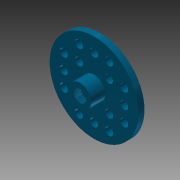
# Autodesk Inventor part: 13-0002
Saved by Autodesk Inventor 2015 SP1 (Build 190203100, 203)
## iProperties
Category: Servo Kit
Company: Autodesk Inc.
Created: 2014-11-30
Part Number: 13-0002
Material: Polystyrene, High Impact
Document SubType Name: Modeling
Designer: Matrix
Density: 1.022 g/cm^3
Appearance: Sky Blue Dark
Catalog Web Link: http://matrixrobotics.com/
Vendor: Matrix
Author: Autodesk Inc.
Autodesk Inventor part; units mm, degrees
ref_plane "YZ Plane" through (0, 0, 0) normal (1, 0, 0) x (0, 1, 0)
ref_plane "XZ Plane" through (0, 0, 0) normal (0, 1, 0) x (-1, 0, 0)
sketch "Sketch1" plane through (0, 0, 0) normal (0, 1, 0) x (-1, 0, 0)
  circle A0 centre (0, 0) radius 6
  circle A1 centre (0, 0) radius 23.5
  circle A2 centre (8, -8) radius 2.1
  circle A3 centre (-8, -8) radius 2.1
  circle A4 centre (7.961966, 8) radius 2.1
  circle A5 centre (-8, 8) radius 2.1
  circle A6 centre (0, 16) radius 2.1
  circle A7 centre (16, 8) radius 2.1
  circle A8 centre (16, -8) radius 2.1
  circle A9 centre (0, -16) radius 2.1
  circle A10 centre (-16, -8) radius 2.1
  circle A11 centre (-16, 8) radius 2.1
  circle A12 centre (0, 0) radius 3
  circle A13 centre (-16, 0) radius 2.1
  circle A14 centre (-8, -16) radius 2.1
  circle A15 centre (8, -16) radius 2.1
  circle A16 centre (16, 0) radius 2.1
  circle A17 centre (8, 16) radius 2.1
  circle A18 centre (-8, 16) radius 2.1
  constraints: 19 centre point
extrude "Extrusion1" add sketch "Sketch1" against normal blind 3.2 contours A0 | A1 | A12
extrude "Extrusion2" add sketch "Sketch1" along normal blind 7.5 contours A0 | A12
sketch "Sketch2" plane through (0, 7.5, 0) normal (0, 1, 0) x (1, 0, 0)
  line L0 (0.096605, 3.117984) -> (0.054534, 3.057901)
  arc A0 (-0.937297, 2.916297) -> (-1.313083, 2.767513) centre (-1.085967, 2.74284) ccw
  line L1 (-0.937297, 2.916297) -> (-0.881604, 2.868563)
  arc A1 (-0.881604, 2.868563) -> (-0.609384, 2.938457) centre (-0.769964, 2.998815) ccw
  line L2 (-0.609384, 2.938457) -> (-0.583576, 3.007117)
  arc A2 (-0.182595, 3.057773) -> (-0.583576, 3.007117) centre (-0.369732, 2.926739) ccw
  line L3 (-0.182595, 3.057773) -> (-0.140524, 2.997689)
  arc A3 (-0.140524, 2.997689) -> (0.140525, 2.997689) centre (0.000001, 3.096085) ccw
  line L4 (0.140525, 2.997689) -> (0.182596, 3.057773)
  arc A4 (0.583577, 3.007117) -> (0.182596, 3.057773) centre (0.369733, 2.926738) ccw
  line L5 (0.583577, 3.007117) -> (0.609385, 2.938457)
  arc A5 (0.609385, 2.938457) -> (0.881605, 2.868563) centre (0.769965, 2.998815) ccw
  line L6 (0.881605, 2.868563) -> (0.937297, 2.916297)
  arc A6 (1.313083, 2.767513) -> (0.937297, 2.916297) centre (1.085967, 2.74284) ccw
  line L7 (1.313083, 2.767513) -> (1.321005, 2.694592)
  arc A7 (1.321005, 2.694592) -> (1.56729, 2.559195) centre (1.49155, 2.713119) ccw
  line L8 (1.56729, 2.559195) -> (1.633105, 2.59158)
  arc A8 (1.960083, 2.354016) -> (1.633105, 2.59158) centre (1.733967, 2.3866) ccw
  line L9 (1.960083, 2.354016) -> (1.949622, 2.281416)
  arc A9 (1.949622, 2.281416) -> (2.154499, 2.089025) centre (2.119417, 2.256948) ccw
  line L10 (2.154499, 2.089025) -> (2.226295, 2.104024)
  arc A10 (2.483923, 1.792608) -> (2.226295, 2.104024) centre (2.273014, 1.880401) ccw
  line L11 (2.483923, 1.792608) -> (2.455735, 1.724891)
  arc A11 (2.455735, 1.724891) -> (2.606329, 1.487593) centre (2.614111, 1.658965) ccw
  line L12 (2.606329, 1.487593) -> (2.679603, 1.484265)
  arc A12 (2.851689, 1.118563) -> (2.679603, 1.484265) centre (2.66924, 1.256049) ccw
  line L13 (2.851689, 1.118563) -> (2.807546, 1.059983)
  arc A13 (2.807546, 1.059983) -> (2.894395, 0.792689) centre (2.944551, 0.956742) ccw
  line L14 (2.894395, 0.792689) -> (2.964538, 0.771244)
  arc A14 (3.040272, 0.374235) -> (2.964538, 0.771244) centre (2.897746, 0.552775) ccw
  line L15 (3.040272, 0.374235) -> (2.982949, 0.328474)
  arc A15 (2.982949, 0.328474) -> (3.000596, 0.047979) centre (3.089974, 0.194405) ccw
  line L16 (3.000596, 0.047979) -> (3.063204, 0.009763)
  arc A16 (3.037826, -0.393607) -> (3.063204, 0.009763) centre (2.944179, -0.185232) ccw
  line L17 (3.037826, -0.393607) -> (2.970922, -0.423676)
  arc A17 (2.970922, -0.423676) -> (2.91826, -0.699748) centre (3.041244, -0.580149) ccw
  line L18 (2.91826, -0.699748) -> (2.969394, -0.75233)
  arc A18 (2.844501, -1.136718) -> (2.969394, -0.75233) centre (2.805617, -0.9116) ccw
  line L19 (2.844501, -1.136718) -> (2.772221, -1.149203)
  arc A19 (2.772221, -1.149203) -> (2.652556, -1.403504) centre (2.80142, -1.318249) ccw
  line L20 (2.652556, -1.403504) -> (2.689009, -1.467155)
  arc A20 (2.472445, -1.808406) -> (2.689009, -1.467155) centre (2.490767, -1.58069) ccw
  line L21 (2.472445, -1.808406) -> (2.399332, -1.802523)
  arc A21 (2.399332, -1.802523) -> (2.220185, -2.019077) centre (2.385574, -1.97352) ccw
  line L22 (2.220185, -2.019077) -> (2.239663, -2.089789)
  arc A22 (1.945037, -2.366463) -> (2.239663, -2.089789) centre (2.019414, -2.150457) ccw
  line L23 (1.945037, -2.366463) -> (1.875683, -2.342582)
  arc A23 (1.875683, -2.342582) -> (1.648309, -2.507782) centre (1.819832, -2.504785) ccw
  line L24 (1.648309, -2.507782) -> (1.64959, -2.581114)
  arc A24 (1.295415, -2.775827) -> (1.64959, -2.581114) centre (1.421174, -2.585104) ccw
  line L25 (1.295415, -2.775827) -> (1.234179, -2.735448)
  arc A25 (1.234179, -2.735448) -> (0.972865, -2.838911) centre (1.139744, -2.878666) ccw
  line L26 (0.972865, -2.838911) -> (0.955868, -2.910262)
  arc A26 (0.564397, -3.010776) -> (0.955868, -2.910262) centre (0.733635, -2.85732) ccw
  line L27 (0.564397, -3.010776) -> (0.515127, -2.956438)
  arc A27 (0.515127, -2.956438) -> (0.236294, -2.991663) centre (0.388043, -3.071671) ccw
  line L28 (0.236294, -2.991663) -> (0.202085, -3.056547)
  arc A28 (-0.202083, -3.056547) -> (0.202085, -3.056547) centre (0.000001, -2.95) ccw
  line L29 (-0.202083, -3.056547) -> (-0.236293, -2.991662)
  arc A29 (-0.236293, -2.991662) -> (-0.515126, -2.956437) centre (-0.388042, -3.07167) ccw
  line L30 (-0.515126, -2.956437) -> (-0.564398, -3.010776)
  arc A30 (-0.955868, -2.910263) -> (-0.564398, -3.010776) centre (-0.733636, -2.85732) ccw
  line L31 (-0.955868, -2.910263) -> (-0.972866, -2.838911)
  arc A31 (-0.972866, -2.838911) -> (-1.23418, -2.73545) centre (-1.139745, -2.878667) ccw
  line L32 (-1.23418, -2.73545) -> (-1.295415, -2.775827)
  arc A32 (-1.64959, -2.581115) -> (-1.295415, -2.775827) centre (-1.421173, -2.585105) ccw
  line L33 (-1.64959, -2.581115) -> (-1.648309, -2.507781)
  arc A33 (-1.648309, -2.507781) -> (-1.875683, -2.342582) centre (-1.819832, -2.504785) ccw
  line L34 (-1.875683, -2.342582) -> (-1.945037, -2.366463)
  arc A34 (-2.239662, -2.089788) -> (-1.945037, -2.366463) centre (-2.019414, -2.150457) ccw
  line L35 (-2.239662, -2.089788) -> (-2.220184, -2.019076)
  arc A35 (-2.220184, -2.019076) -> (-2.399331, -1.802522) centre (-2.385573, -1.973519) ccw
  line L36 (-2.399331, -1.802522) -> (-2.472446, -1.808405)
  arc A36 (-2.68901, -1.467155) -> (-2.472446, -1.808405) centre (-2.490767, -1.580689) ccw
  line L37 (-2.68901, -1.467155) -> (-2.652557, -1.403504)
  arc A37 (-2.652557, -1.403504) -> (-2.772222, -1.149203) centre (-2.801421, -1.318249) ccw
  line L38 (-2.772222, -1.149203) -> (-2.844501, -1.136718)
  arc A38 (-2.969396, -0.752332) -> (-2.844501, -1.136718) centre (-2.805617, -0.9116) ccw
  line L39 (-2.969396, -0.752332) -> (-2.918259, -0.699746)
  arc A39 (-2.918259, -0.699746) -> (-2.970923, -0.423675) centre (-3.041244, -0.580148) ccw
  line L40 (-2.970923, -0.423675) -> (-3.037826, -0.393607)
  arc A40 (-3.063204, 0.009763) -> (-3.037826, -0.393607) centre (-2.944179, -0.185232) ccw
  line L41 (-3.063204, 0.009763) -> (-3.000596, 0.047979)
  arc A41 (-3.000596, 0.047979) -> (-2.982949, 0.328474) centre (-3.089974, 0.194405) ccw
  line L42 (-2.982949, 0.328474) -> (-3.040274, 0.374236)
  arc A42 (-2.96454, 0.771245) -> (-3.040274, 0.374236) centre (-2.897747, 0.552776) ccw
  line L43 (-2.96454, 0.771245) -> (-2.894397, 0.79269)
  arc A43 (-2.894397, 0.79269) -> (-2.807548, 1.059984) centre (-2.944553, 0.956743) ccw
  line L44 (-2.807548, 1.059984) -> (-2.85169, 1.118562)
  arc A44 (-2.679604, 1.484265) -> (-2.85169, 1.118562) centre (-2.66924, 1.256048) ccw
  line L45 (-2.679604, 1.484265) -> (-2.606328, 1.487592)
  arc A45 (-2.606328, 1.487592) -> (-2.455735, 1.72489) centre (-2.61411, 1.658964) ccw
  line L46 (-2.455735, 1.72489) -> (-2.483923, 1.792608)
  arc A46 (-2.226297, 2.104025) -> (-2.483923, 1.792608) centre (-2.273014, 1.880401) ccw
  line L47 (-2.226297, 2.104025) -> (-2.154496, 2.089025)
  arc A47 (-2.154496, 2.089025) -> (-1.94962, 2.281418) centre (-2.119415, 2.256948) ccw
  line L48 (-1.94962, 2.281418) -> (-1.960082, 2.354014)
  arc A48 (-1.633104, 2.59158) -> (-1.960082, 2.354014) centre (-1.733966, 2.3866) ccw
  line L49 (-1.633104, 2.59158) -> (-1.56729, 2.559196)
  arc A49 (-1.56729, 2.559196) -> (-1.321004, 2.694592) centre (-1.49155, 2.71312) ccw
  line L50 (-1.321004, 2.694592) -> (-1.313083, 2.767513)
  point P0 (0, 0)
  point P1 (0, 0)
  point P2 (0, 0)
  constraints: 102 end point, 100 point on circle, 50 centre point
ref_plane "Work Plane1" through (0, 4, 0) normal (0, 1, 0) x (1, 0, 0)
sketch "Sketch5" plane through (0, 4, 0) normal (0, 1, 0) x (1, 0, 0)
  circle A0 centre (0, 0) radius 3
  arc A1 (0.416534, 2.94433) -> (0.328774, 2.955416) centre (0.369731, 2.926738) ccw
  line L0 (0.328774, 2.955416) -> (0.286701, 2.895331)
  arc A2 (-0.286705, 2.895331) -> (0.286701, 2.895331) centre (-0.000002, 3.096083) ccw
  line L1 (-0.286705, 2.895331) -> (-0.328778, 2.955417)
  arc A3 (-0.328778, 2.955417) -> (-0.416538, 2.94433) centre (-0.369735, 2.926738) ccw
  line L2 (-0.416538, 2.94433) -> (-0.442346, 2.875669)
  arc A4 (-0.997737, 2.733069) -> (-0.442346, 2.875669) centre (-0.769966, 2.998814) ccw
  line L3 (-0.997737, 2.733069) -> (-1.053431, 2.780803)
  arc A5 (-1.053431, 2.780803) -> (-1.135677, 2.74824) centre (-1.085969, 2.74284) ccw
  line L4 (-1.143599, 2.675318) -> (-1.135677, 2.74824)
  arc A6 (-1.646079, 2.399078) -> (-1.143599, 2.675318) centre (-1.491551, 2.713118) ccw
  line L5 (-1.646079, 2.399078) -> (-1.711893, 2.431462)
  arc A7 (-1.711893, 2.431462) -> (-1.783457, 2.379469) centre (-1.733968, 2.386599) ccw
  line L6 (-1.772995, 2.306867) -> (-1.783457, 2.379469)
  arc A8 (-2.19099, 1.914343) -> (-1.772995, 2.306867) centre (-2.119417, 2.256947) ccw
  line L7 (-2.262791, 1.929343) -> (-2.19099, 1.914343)
  arc A9 (-2.262791, 1.929343) -> (-2.319345, 1.861595) centre (-2.273016, 1.8804) ccw
  line L8 (-2.319345, 1.861595) -> (-2.290986, 1.793468)
  arc A10 (-2.598233, 1.309325) -> (-2.290986, 1.793468) centre (-2.61411, 1.658965) ccw
  line L9 (-2.671508, 1.305997) -> (-2.598233, 1.309325)
  arc A11 (-2.671508, 1.305997) -> (-2.709172, 1.225958) centre (-2.66924, 1.256049) ccw
  line L10 (-2.709172, 1.225958) -> (-2.665028, 1.167378)
  arc A12 (-2.84222, 0.622036) -> (-2.665028, 1.167378) centre (-2.94455, 0.956742) ccw
  line L11 (-2.912366, 0.60059) -> (-2.84222, 0.622036)
  arc A13 (-2.912366, 0.60059) -> (-2.928941, 0.513699) centre (-2.897747, 0.552775) ccw
  line L12 (-2.928941, 0.513699) -> (-2.871616, 0.467937)
  arc A14 (-2.907621, -0.104338) -> (-2.871616, 0.467937) centre (-3.089974, 0.194405) ccw
  line L13 (-2.907621, -0.104338) -> (-2.970229, -0.142554)
  arc A15 (-2.970229, -0.142554) -> (-2.964676, -0.230838) centre (-2.944179, -0.185232) ccw
  line L14 (-2.964676, -0.230838) -> (-2.89777, -0.260906)
  arc A16 (-2.790325, -0.824156) -> (-2.89777, -0.260906) centre (-3.041243, -0.580148) ccw
  line L15 (-2.790325, -0.824156) -> (-2.841462, -0.876742)
  arc A17 (-2.841462, -0.876742) -> (-2.814127, -0.960871) centre (-2.805617, -0.9116) ccw
  line L16 (-2.741847, -0.973356) -> (-2.814127, -0.960871)
  arc A18 (-2.497702, -1.492189) -> (-2.741847, -0.973356) centre (-2.80142, -1.318248) ccw
  line L17 (-2.497702, -1.492189) -> (-2.534156, -1.55584)
  arc A19 (-2.534156, -1.55584) -> (-2.486757, -1.630528) centre (-2.490767, -1.580689) ccw
  line L18 (-2.413643, -1.624645) -> (-2.486757, -1.630528)
  arc A20 (-2.04814, -2.066463) -> (-2.413643, -1.624645) centre (-2.385573, -1.973518) ccw
  line L19 (-2.067619, -2.137179) -> (-2.04814, -2.066463)
  arc A21 (-2.067619, -2.137179) -> (-2.003136, -2.197733) centre (-2.019414, -2.150457) ccw
  line L20 (-1.933781, -2.173853) -> (-2.003136, -2.197733)
  arc A22 (-1.469886, -2.510891) -> (-1.933781, -2.173853) centre (-1.819832, -2.504784) ccw
  line L21 (-1.471166, -2.584233) -> (-1.469886, -2.510891)
  arc A23 (-1.471166, -2.584233) -> (-1.393649, -2.626847) centre (-1.421173, -2.585105) ccw
  line L22 (-1.393649, -2.626847) -> (-1.332413, -2.586469)
  arc A24 (-0.799273, -2.797554) -> (-1.332413, -2.586469) centre (-1.139744, -2.878666) ccw
  line L23 (-0.782274, -2.868908) -> (-0.799273, -2.797554)
  arc A25 (-0.782274, -2.868908) -> (-0.696595, -2.890906) centre (-0.733635, -2.85732) ccw
  line L24 (-0.696595, -2.890906) -> (-0.647324, -2.836568)
  arc A26 (-0.078439, -2.908435) -> (-0.647324, -2.836568) centre (-0.388042, -3.07167) ccw
  line L25 (-0.078439, -2.908435) -> (-0.044229, -2.973319)
  arc A27 (-0.044229, -2.973319) -> (0.044229, -2.973319) centre (0, -2.95) ccw
  line L26 (0.044229, -2.973319) -> (0.078439, -2.908435)
  arc A28 (0.647324, -2.836568) -> (0.078439, -2.908435) centre (0.388042, -3.07167) ccw
  line L27 (0.647324, -2.836568) -> (0.696595, -2.890906)
  arc A29 (0.696595, -2.890906) -> (0.782274, -2.868908) centre (0.733635, -2.85732) ccw
  line L28 (0.799273, -2.797554) -> (0.782274, -2.868908)
  arc A30 (1.332413, -2.586469) -> (0.799273, -2.797554) centre (1.139744, -2.878666) ccw
  line L29 (1.332413, -2.586469) -> (1.39365, -2.626847)
  arc A31 (1.39365, -2.626847) -> (1.471173, -2.585105) centre (1.421173, -2.585105) ccw
  line L30 (1.469771, -2.504785) -> (1.471173, -2.585105)
  arc A32 (1.93372, -2.173854) -> (1.469771, -2.504785) centre (1.819771, -2.504785) ccw
  line L31 (2.003075, -2.197734) -> (1.93372, -2.173854)
  arc A33 (2.003075, -2.197734) -> (2.067558, -2.137181) centre (2.019353, -2.150458) ccw
  line L32 (2.048079, -2.066464) -> (2.067558, -2.137181)
  arc A34 (2.413582, -1.624646) -> (2.048079, -2.066464) centre (2.385512, -1.973519) ccw
  line L33 (2.486697, -1.630529) -> (2.413582, -1.624646)
  arc A35 (2.486697, -1.630529) -> (2.534095, -1.555841) centre (2.490706, -1.58069) ccw
  line L34 (2.534095, -1.555841) -> (2.497641, -1.49219)
  arc A36 (2.741786, -0.973357) -> (2.497641, -1.49219) centre (2.801359, -1.318249) ccw
  line L35 (2.814066, -0.960872) -> (2.741786, -0.973357)
  arc A37 (2.814066, -0.960872) -> (2.841402, -0.876743) centre (2.805556, -0.911601) ccw
  line L36 (2.841402, -0.876743) -> (2.790264, -0.824157)
  arc A38 (2.897709, -0.260907) -> (2.790264, -0.824157) centre (3.041183, -0.580149) ccw
  line L37 (2.897709, -0.260907) -> (2.964614, -0.230839)
  arc A39 (2.964614, -0.230839) -> (2.970168, -0.142556) centre (2.944118, -0.185233) ccw
  line L38 (2.970168, -0.142556) -> (2.90756, -0.104339)
  arc A40 (2.871615, 0.467936) -> (2.90756, -0.104339) centre (3.089947, 0.194383) ccw
  line L39 (2.871615, 0.467936) -> (2.92894, 0.513698)
  arc A41 (2.92894, 0.513698) -> (2.912363, 0.60059) centre (2.897746, 0.552774) ccw
  line L40 (2.842219, 0.622035) -> (2.912363, 0.60059)
  arc A42 (2.665026, 1.167377) -> (2.842219, 0.622035) centre (2.944549, 0.956742) ccw
  line L41 (2.665026, 1.167377) -> (2.709169, 1.225957)
  arc A43 (2.709169, 1.225957) -> (2.671506, 1.305997) centre (2.669238, 1.256048) ccw
  line L42 (2.598231, 1.309324) -> (2.671506, 1.305997)
  arc A44 (2.290984, 1.793467) -> (2.598231, 1.309324) centre (2.614108, 1.658964) ccw
  line L43 (2.290984, 1.793467) -> (2.319173, 1.861185)
  arc A45 (2.319173, 1.861185) -> (2.262787, 1.929343) centre (2.273012, 1.8804) ccw
  line L44 (2.190987, 1.914343) -> (2.262787, 1.929343)
  arc A46 (1.772992, 2.306867) -> (2.190987, 1.914343) centre (2.119413, 2.256947) ccw
  line L45 (1.783454, 2.37947) -> (1.772992, 2.306867)
  arc A47 (1.783454, 2.37947) -> (1.711889, 2.431462) centre (1.733965, 2.386599) ccw
  line L46 (1.711889, 2.431462) -> (1.646075, 2.399078)
  arc A48 (1.143595, 2.675318) -> (1.646075, 2.399078) centre (1.491548, 2.713118) ccw
  line L47 (1.135673, 2.748239) -> (1.143595, 2.675318)
  arc A49 (1.135673, 2.748239) -> (1.053427, 2.780803) centre (1.085966, 2.74284) ccw
  line L48 (1.053427, 2.780803) -> (0.997734, 2.733069)
  arc A50 (0.442342, 2.875669) -> (0.997734, 2.733069) centre (0.769963, 2.998814) ccw
  line L49 (0.442342, 2.875669) -> (0.416534, 2.94433)
  circle A51 centre (0, 0) radius 1.25
  constraints: 100 end point, 100 point on circle, 52 centre point
extrude "Extrusion3" cut sketch "Sketch2" against normal blind 3.5 draft -2.5
sketch "Sketch6" plane through (0, -3.2, 0) normal (0, -1, 0) x (1, 0, 0)
  circle A0 centre (0, 0) radius 3
  dimension "d7" = 6
  constraints: 1 centre point, 1 coincident
  measures "d7" diameter of A0
extrude "Extrusion4" cut sketch "Sketch6" against normal blind 6.2
extrude "Extrusion5" cut sketch "Sketch5" against normal through all contours A51
chamfer "Chamfer1" distance 0.1 angle 45 100 edges at (1.1701, 7.5, -2.9552) (1.317, 7.5, -2.7311) (1.4089, 7.5, -2.5628) (1.6002, 7.5, -2.5754) (1.8682, 7.5, -2.5714) (1.9549, 7.5, -2.3177) (2.002, 7.5, -2.1319) (2.1904, 7.5, -2.0965) (2.449, 7.5, -2.026) (2.4698, 7.5, -1.7587) (2.4693, 7.5, -1.567) (2.643, 7.5, -1.4859) (2.8759, 7.5, -1.3533) (2.8296, 7.5, -1.0893) (2.7814, 7.5, -0.9037) (2.9295, 7.5, -0.782) (3.1222, 7.5, -0.5956) (3.0116, 7.5, -0.3514) (2.9188, 7.5, -0.1836) (3.0319, 7.5, -0.0289) (3.1722, 7.5, 0.1996) (3.0044, 7.5, 0.4086) (2.8727, 7.5, 0.548) (2.9438, 7.5, 0.726) (3.0229, 7.5, 0.9822) (2.8084, 7.5, 1.143) (2.6462, 7.5, 1.2452) (2.6708, 7.5, 1.4353) (2.6837, 7.5, 1.7031) (2.4359, 7.5, 1.8055) (2.2534, 7.5, 1.8642) (2.2299, 7.5, 2.0544) (2.1758, 7.5, 2.317) (1.9104, 7.5, 2.3545) (1.719, 7.5, 2.366) (1.6489, 7.5, 2.5444) (1.5312, 7.5, 2.7853) (1.2648, 7.5, 2.7556) (1.0766, 7.5, 2.7192) (0.9644, 7.5, 2.8746) (0.7904, 7.5, 3.0786) (0.5398, 7.5, 2.9836) (0.3665, 7.5, 2.9015) (0.2192, 7.5, 3.0241) (0, 7.5, 3.1785) (-0.2192, 7.5, 3.0241) (-0.3665, 7.5, 2.9015) (-0.5398, 7.5, 2.9836) (-0.7904, 7.5, 3.0786) (-0.9644, 7.5, 2.8746) (-1.0766, 7.5, 2.7192) (-1.2648, 7.5, 2.7556) (-1.5312, 7.5, 2.7853) (-1.6489, 7.5, 2.5444) (-1.719, 7.5, 2.366) (-1.9104, 7.5, 2.3545) (-2.1758, 7.5, 2.317) (-2.2299, 7.5, 2.0544) (-2.2534, 7.5, 1.8642) (-2.4359, 7.5, 1.8055) (-2.6837, 7.5, 1.7031) (-2.6708, 7.5, 1.4353) (-2.6462, 7.5, 1.2452) (-2.8084, 7.5, 1.143) (-3.0229, 7.5, 0.9822) (-2.9438, 7.5, 0.726) (-2.8727, 7.5, 0.548) (-3.0044, 7.5, 0.4086) (-3.1722, 7.5, 0.1996) (-3.0319, 7.5, -0.0289) (-2.9188, 7.5, -0.1836) (-3.0116, 7.5, -0.3514) (-3.1222, 7.5, -0.5956) (-2.9295, 7.5, -0.782) (-2.7814, 7.5, -0.9037) (-2.8296, 7.5, -1.0893) (-2.8759, 7.5, -1.3533) (-2.643, 7.5, -1.4859) (-2.4693, 7.5, -1.567) (-2.4698, 7.5, -1.7587) (-2.449, 7.5, -2.026) (-2.1904, 7.5, -2.0965) (-2.002, 7.5, -2.1319) (-1.9549, 7.5, -2.3177) (-1.8682, 7.5, -2.5714) (-1.6002, 7.5, -2.5754) (-1.4089, 7.5, -2.5628) (-1.317, 7.5, -2.7311) (-1.1701, 7.5, -2.9552) (-0.9095, 7.5, -2.8924) (-0.7273, 7.5, -2.8327) (-0.5965, 7.5, -2.9728) (-0.3984, 7.5, -3.1534) (-0.1616, 7.5, -3.0277) (0, 7.5, -2.9245) (0.1616, 7.5, -3.0277) (0.3984, 7.5, -3.1534) (0.5965, 7.5, -2.9728) (0.7273, 7.5, -2.8327) (0.9095, 7.5, -2.8924)
body "Solid1"
